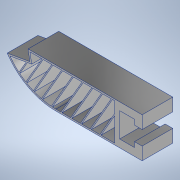
# Autodesk Inventor part: Finray_9_Kerbe_10deg_20deg10inf_PLA
Saved by Autodesk Inventor 2022 (Build 260153000, 153)
## iProperties
Created: 2022-02-28
Part Number: Finray_9_Kerbe_10deg_20deg10inf_PLA
Material: Generic
Document SubType Name: Modeling
Designer: richa
Density: 1 g/cm^3
Appearance: Aluminum - Flat
Author: richa
Autodesk Inventor part; units mm, degrees
ref_plane "YZ Plane" through (0, 0, 0) normal (1, 0, 0) x (0, 1, 0)
ref_plane "XZ Plane" through (0, 0, 0) normal (0, 1, 0) x (-1, 0, 0)
ref_plane "XY Plane" through (0, 0, 0) normal (0, 0, 1) x (1, 0, 0)
sketch "Sketch5" plane through (0, 0, 0) normal (0, 0, 1) x (1, 0, 0)
  line L0 (52.8, -15.6) -> (52.8, -10.6)
  line L1 (52.8, -10.6) -> (49.8, -10.6)
  line L2 (49.8, -10.6) -> (49.8, -12.6)
  line L3 (44, -12.6) -> (44, -3)
  line L4 (49.8, -3) -> (49.8, -5)
  line L5 (49.8, -5) -> (52.8, -5)
  line L6 (52.8, -5) -> (52.8, 0)
  line L7 (52.8, 0) -> (7.8, 0)
  line L8 (44, -3) -> (49.8, -3)
  line L9 (44, -12.6) -> (49.8, -12.6)
  line L10 (52.8, -15.6) -> (7.8, -15.6)
  line L11 (7.8, -15.6) -> (0, -15.6)
  line L12 (0, -15.6) -> (0, 0)
  line L13 (0, 0) -> (7.8, 0)
  point P0 (7.8, 0)
  dimension "d41" = 5.8
  dimension "d48" = 44
  dimension "d50" = 3
  dimension "d63" = 45
  dimension "d71" = 0
  dimension "d87" = 5.6
  dimension "d88" = 9.6
  dimension "d97" = 15.6
  constraints: 28 end point, 8 perpendicular, 4 collinear, 3 parallel, 2 horizontal, 1 vertical
  measures "d41" distance between parallel lines of L2 L3
  measures "d48" distance from line of L3 L12.end
  measures "d50" distance of L4.end L5.end
  measures "d63" distance of L0.start L10.end
  measures "d71" distance from line of L12.end L7
  measures "d87" distance from line of L0.end L5
  measures "d88" distance of L3.start L3.end
  measures "d97" distance of L11.end L12.end
extrude "Extrusion2" add sketch "Sketch5" along normal blind 12
sketch "Sketch8" plane through (0, 0, 0) normal (0, 0, -1) x (-1, 0, 0)
  line L0 (-8.1687, 0) -> (-8.8633, -3.9392)
  line L1 (-7.8, 0) -> (-1.143, 0) construction
  line L2 (0, -5.5021) -> (-8.8633, -3.9392)
  line L3 (-7.8, 0) -> (-8.1687, 0)
  line L4 (0, 0) -> (0, -15.6) projected
  line L5 (-52.8, 0) -> (0, 0) projected
  line L6 (-7.8, 0) -> (0, 0)
  line L7 (0, 0) -> (0, -5.5021)
  dimension "d80" = 100
  dimension "d95" = 4
  dimension "d96" = 9
  constraints: 12 end point, 2 collinear, 2 perpendicular, 1 horizontal, 1 point on line
  measures "d80" angle of L0 L1
  measures "d95" distance of L0.start L0.end
  measures "d96" distance of L2.start L0.end
extrude "Extrusion5" cut sketch "Sketch8" against normal through all
fillet "Fillet2" radius 23 1 edges at (0, -15.6, 6)
shell "Shell1" thickness 0.62 removed faces 1 at (23.9679, -7.5131, 12)
sketch "Sketch13" plane through (0, 0, 12) normal (0, 0, 1) x (1, 0, 0)
  line L0 (19.0404, -15.6) -> (52.8, -15.6) projected
  line L1 (42.0526, -15.6) -> (42.0526, 0)
  line L2 (52.8, 0) -> (8.1687, 0) projected
  line L3 (52.8, 0) -> (8.1687, 0) projected
  line L4 (52.8, -5) -> (52.8, 0) projected
  line L5 (49.8, -5) -> (52.8, -5) projected
  line L6 (49.8, -3) -> (49.8, -5) projected
  line L7 (44, -3) -> (49.8, -3) projected
  line L8 (44, -12.6) -> (44, -3) projected
  line L9 (49.8, -12.6) -> (44, -12.6) projected
  line L10 (49.8, -10.6) -> (49.8, -12.6) projected
  line L11 (52.8, -10.6) -> (49.8, -10.6) projected
  line L12 (52.8, -15.6) -> (52.8, -10.6) projected
  line L13 (42.0526, 0) -> (52.8, 0)
  line L14 (52.8, -5) -> (52.8, 0) projected
  line L15 (52.8, -5) -> (52.8, 0)
  line L16 (52.8, 0) -> (52.8, -5)
  line L17 (44, -12.6) -> (44, -3) projected
  line L18 (44, -3) -> (44, -12.6)
  line L19 (49.8, -12.6) -> (44, -12.6) projected
  line L20 (44, -12.6) -> (49.8, -12.6)
  line L21 (43.38, -13.22) -> (50.42, -13.22) projected
  line L22 (52.8, -10.6) -> (52.8, -15.6)
  line L23 (52.8, -15.6) -> (42.0526, -15.6)
  line L24 (44, -3) -> (49.8, -3) projected
  line L25 (44, -3) -> (49.8, -3)
  line L26 (49.8, -3) -> (49.8, -5)
  line L27 (49.8, -5) -> (52.8, -5)
  line L28 (52.8, -10.6) -> (49.8, -10.6)
  line L29 (49.8, -10.6) -> (49.8, -12.6)
  point P0 (0, 0)
  dimension "d102" = 10.7474
  constraints: 26 end point, 10 collinear, 2 point on line, 2 vertical, 1 parallel
  measures "d102" distance between parallel lines of L4 L1
extrude "Extrusion7" add sketch "Sketch13" against normal blind 12
sketch "Sketch14" plane through (8.9076, -0.62, 0.62) normal (0, 0, 1) x (1, 0, 0)
  line L0 (33.145, -14.36) -> (33.145, 0) projected
  line L1 (33.145, 0) -> (0, 0) projected
  line L2 (0.6739, -3.8221) -> (0, 0) projected
  line L3 (-7.835, -5.3225) -> (0.6739, -3.8221) projected
  arc A0 (-7.835, -5.3225) -> (10.1328, -14.36) centre (10.1328, 8.02) ccw projected
  line L4 (10.1328, -14.36) -> (33.145, -14.36) projected
  point P0 (-8.9076, 0.62)
extrude "Extrusion8" cut sketch "Sketch14" against normal blind 12
sketch "Sketch15" plane through (0, 0, 12) normal (0, 0, 1) x (1, 0, 0)
  line L0 (42.0526, -0.62) -> (8.9076, -0.62) construction
  line L1 (19.0404, -14.98) -> (42.0526, -14.98) projected
  line L2 (44.6611, -0.43) -> (44.9902, -0.62)
  line L3 (44.9902, -0.62) -> (36.5897, -15.17)
  line L4 (36.5897, -15.17) -> (36.2606, -14.98)
  line L5 (36.2606, -14.98) -> (44.6611, -0.43)
  arc A0 (1.0726, -5.9425) -> (19.0404, -14.98) centre (19.0404, 7.4) ccw projected
  line L6 (42.0526, -0.62) -> (42.0526, -14.98) projected
  line L7 (1.0726, -5.9425) -> (9.5815, -4.4421) projected
  arc A1 (0, -5.5021) -> (19.0404, -15.6) centre (19.0404, 7.4) ccw projected
  line L8 (42.0526, -14.98) -> (19.0404, -14.98) projected
  line L9 (8.9076, -0.62) -> (42.0526, -0.62) projected
  line L10 (41.1802, -0.62) -> (32.8894, -14.98)
  line L11 (40.7414, -0.62) -> (32.4506, -14.98)
  line L12 (33.5602, -0.62) -> (25.2694, -14.98)
  line L13 (33.1214, -0.62) -> (24.8306, -14.98)
  line L14 (29.7502, -0.62) -> (21.4594, -14.98)
  line L15 (29.3114, -0.62) -> (21.0206, -14.98)
  line L16 (25.9402, -0.62) -> (17.6494, -14.98)
  line L17 (25.5014, -0.62) -> (17.2106, -14.98)
  line L18 (21.7132, -0.62) -> (13.7839, -14.3539)
  line L19 (17.9032, -0.62) -> (10.5729, -13.3163)
  line L20 (17.4644, -0.62) -> (10.2196, -13.1684)
  line L21 (14.0932, -0.62) -> (7.6136, -11.843)
  line L22 (13.6544, -0.62) -> (7.2884, -11.6462)
  line L23 (10.2832, -0.62) -> (4.8989, -9.9459)
  line L24 (9.8444, -0.62) -> (4.6022, -9.6998)
  line L25 (21.2744, -0.62) -> (13.4006, -14.2577)
  line L26 (37.3702, -0.62) -> (29.0794, -14.98)
  line L27 (36.9314, -0.62) -> (28.6406, -14.98)
  line L28 (8.9076, -0.62) -> (0, -0.62) construction
  point P0 (0, 0)
  point P1 (36.2606, -14.98)
  point P2 (7.9059, -4.7376)
  point P3 (7.4174, -4.8237)
  point P4 (36.6994, -14.98)
  point P5 (36.2606, -14.98)
  point P6 (32.8894, -14.98)
  point P7 (28.6406, -14.98)
  point P8 (29.0794, -14.98)
  point P9 (25.2694, -14.98)
  point P10 (21.4594, -14.98)
  point P11 (19.1926, -14.98)
  point P12 (19.6314, -14.98)
  point P13 (17.252, -14.9084)
  point P14 (17.6736, -14.9382)
  dimension "d105" = 0.38
  dimension "d130" = 120
  dimension "d132" = 120
  dimension "d133" = 0.38
  dimension "d135" = 0.38
  dimension "d136" = 0.38
  dimension "d137" = 0.38
  dimension "d138" = 0.38
  dimension "d139" = 0.38
  dimension "d140" = 0.38
  dimension "d141" = 0.38
  dimension "d142" = 3.81
  dimension "d143" = 0.38
  dimension "d144" = 3.81
  dimension "d145" = 3.81
  dimension "d146" = 3.81
  dimension "d147" = 3.81
  dimension "d148" = 3.81
  dimension "d152" = 120
  dimension "d153" = 3.81
  dimension "d154" = 3.81
  dimension "d155" = 3.81
  constraints: 46 end point, 18 parallel, 5 point on line, 1 horizontal, 1 perpendicular, 40 other
  measures "d105" distance between parallel lines of L3 L5
  measures "d130" angle of L0 L3
  measures "d132" angle of L0 L10
  measures "d133" distance between parallel lines of L10 L11
  measures "d135" distance between parallel lines of L13 L12
  measures "d136" distance between parallel lines of L15 L14
  measures "d137" distance between parallel lines of L17 L16
  measures "d138" distance between parallel lines of L25 L18
  measures "d139" distance between parallel lines of L20 L19
  measures "d140" distance between parallel lines of L22 L21
  measures "d141" distance between parallel lines of L24 L23
  measures "d142" distance of L4.end L11.end
  measures "d143" distance between parallel lines of L26 L27
  measures "d144" distance of L11.end L27.end
  measures "d145" distance of L27.end L13.end
  measures "d146" distance of L15.end L13.end
  measures "d147" distance of L15.end L17.end
  measures "d148" horizontal distance of L25.end L17.end
  measures "d152" angle of L0 L12
  measures "d153" distance of L22.start L20.start
  measures "d154" distance of L20.start L25.start
  measures "d155" distance of L24.start L22.start
extrude "Extrusion9" add sketch "Sketch15" against normal blind 12 contours L15 L9 L14 L1 | A0 L17 L9 L16 | L13 L9 L12 L1 | A0 L25 L9 L18 | L27 L9 L26 L1 | A0 L20 L9 L19 | L11 L9 L10 L1 | A0 L22 L9 L21 | L5 L6 L3 L1 | A0 L24 L7 L23 | L5 L2 L3 L6
equation "\"l1\" = 8"
equation "\"d1\" = 0.38"
body "Solid2"
